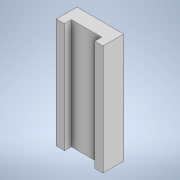
# Autodesk Inventor part: trafficlysidod
Saved by Autodesk Inventor 2022.1 (Build 261234020, 234B)
## iProperties
Created: 2022-01-15
Part Number: trafficlysidod
Material: Generic
Document SubType Name: Modeling
Designer: 46734
Density: 1 g/cm^3
Appearance: Default
Author: 46734
Autodesk Inventor part; units mm, degrees
ref_plane "YZ Plane" through (0, 0, 0) normal (1, 0, 0) x (0, 1, 0)
ref_plane "XZ Plane" through (0, 0, 0) normal (0, 1, 0) x (-1, 0, 0)
ref_plane "XY Plane" through (0, 0, 0) normal (0, 0, 1) x (1, 0, 0)
sketch "Sketch1" plane through (0, 0, 0) normal (0, 0, 1) x (1, 0, 0)
  line L0 (-8.5, 20) -> (8.5, 20)
  line L1 (8.5, 20) -> (8.5, -20)
  line L2 (8.5, -20) -> (-8.5, -20)
  line L3 (-8.5, -20) -> (-8.5, 20)
  line L4 (-8.5, 20) -> (8.5, -20) construction
  line L5 (8.5, 20) -> (-8.5, -20) construction
  point P0 (0, 0)
  dimension "d0" = 17
  dimension "d1" = 40
  constraints: 12 end point, 2 midpoint, 2 parallel, 1 horizontal, 1 perpendicular
  measures "d0" distance of L1.end L2.end
  measures "d1" distance of L0.end L1.end
extrude "Extrusion1" add sketch "Sketch1" along normal blind 5
sketch "Sketch2" plane through (-8.5, -20, 0) normal (0, -1, 0) x (1, 0, 0)
  line L0 (0, 5) -> (17, 5) projected
  line L1 (0, 5) -> (0, 15)
  line L2 (0, 15) -> (17, 15)
  line L3 (17, 15) -> (17, 5)
  line L4 (3, 5) -> (3, 10)
  line L5 (3, 10) -> (14, 10)
  line L6 (14, 10) -> (14, 5)
  point P0 (8.5, 0)
  point P1 (14, 7.5)
  dimension "d4" = 10
  dimension "d12" = 5
  dimension "d13" = 3
  dimension "d14" = 3
  constraints: 12 end point, 4 perpendicular, 2 point on line, 2 vertical, 1 midpoint
  measures "d4" distance of L0.start L1.end
  measures "d12" distance between parallel lines of L5 L2
  measures "d13" distance from line of L3 point (14, 7.5)
  measures "d14" distance between parallel lines of L1 L4
extrude "Extrusion2" add sketch "Sketch2" against normal up to surface (40 mm away) contours L1 L2 L3 L0 L6 L5 L4
sketch "Sketch3" plane through (-8.5, 20, 0) normal (0, 1, 0) x (1, 0, 0)
  line L0 (0, 0) -> (0, -15) projected
  line L1 (0, -7.5) -> (35.2225, -7.5)
  line L2 (35.2225, -7.5) -> (35.2225, -20.6819)
  line L3 (35.2225, -20.6819) -> (0, -20.6819)
  line L4 (0, -20.6819) -> (0, -7.5)
  point P0 (8.5, 0)
  constraints: 8 end point, 2 parallel, 1 horizontal, 1 midpoint, 1 perpendicular
extrude "Extrusion3" cut sketch "Sketch3" against normal through all
body "Solid1"
